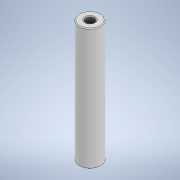
# Autodesk Inventor part: ARL-445KE
Saved by Autodesk Inventor 2022 (Build 260153000, 153)
## iProperties
Created: 2022-03-25
Part Number: ARL-445KE
Material: 一般
Document SubType Name: Modeling
Designer: masayuki
Density: 1 g/cm^3
Appearance: 既定
Author: masayuki
Autodesk Inventor part; units mm, degrees
ref_plane "YZ Plane" through (0, 0, 0) normal (1, 0, 0) x (0, 1, 0)
ref_plane "XZ Plane" through (0, 0, 0) normal (0, 1, 0) x (-1, 0, 0)
ref_plane "XY Plane" through (0, 0, 0) normal (0, 0, 1) x (1, 0, 0)
sketch "スケッチ1" plane through (0, 0, 0) normal (0, 1, 0) x (-1, 0, 0)
  circle A0 centre (0, 0) radius 4
  dimension "d0" = 8
  constraints: 1 centre point, 1 coincident
  measures "d0" diameter of A0
extrude "押し出し1" add sketch "スケッチ1" along normal blind 45
sketch "スケッチ2" plane through (0, 45, 0) normal (0, 1, 0) x (1, 0, 0)
  circle A0 centre (0, 0) radius 1.65
  dimension "d3" = 3.3
  constraints: 1 centre point, 1 coincident
  measures "d3" diameter of A0
extrude "押し出し2" cut sketch "スケッチ2" against normal blind 8
thread "ねじ1" size "M4x0.7" class "6H" standard "ISO Metric profile" full length
sketch "スケッチ3" plane through (0, 0, 0) normal (0, -1, 0) x (1, 0, 0)
  circle A0 centre (0, 0) radius 1.65
  dimension "d8" = 3.3
  constraints: 1 centre point, 1 coincident
  measures "d8" diameter of A0
extrude "押し出し3" cut sketch "スケッチ3" against normal blind 8
thread "ねじ2" size "M4x0.7" class "6H" standard "ISO Metric profile" full length
fillet "フィレット1" radius 0.3 1 edges at (-1.65, 0, 0)
fillet "フィレット2" radius 0.3 1 edges at (-1.65, 45, 0)
fillet "フィレット3" radius 0.3 2 edges at (4, 45, 0) (4, 0, 0)
